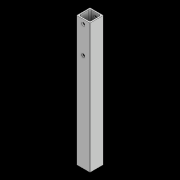
# Autodesk Inventor part: am-3594 5-8x5-8 0.063 wall tubing
Saved by Autodesk Inventor 2022 (Build 260153000, 153)
## iProperties
Created: 2021-10-09
Part Number: am-3594 5-8x5-8 0.063 wall tubing
Material: Generic
Document SubType Name: Modeling
Designer: timmy
Density: 1 g/cm^3
Appearance: Default
Author: timmy
Autodesk Inventor part; units mm, degrees
ref_plane "YZ Plane" through (0, 0, 0) normal (1, 0, 0) x (0, 1, 0)
ref_plane "XZ Plane" through (0, 0, 0) normal (0, 1, 0) x (-1, 0, 0)
ref_plane "XY Plane" through (0, 0, 0) normal (0, 0, 1) x (1, 0, 0)
sketch "Sketch1" plane through (0, 0, 0) normal (0, 1, 0) x (-1, 0, 0)
  line L0 (0, 0) -> (-15.875, 0)
  line L1 (-15.875, 0) -> (-15.875, -15.875)
  line L2 (-15.875, -15.875) -> (0, -15.875)
  line L3 (0, -15.875) -> (0, 0)
  dimension "d0" = 15.875
  dimension "d1" = 15.875
  constraints: 8 end point, 2 parallel, 1 horizontal, 1 perpendicular
  measures "d0" distance of L2.end L1.end
  measures "d1" distance of L1.end L0.end
extrude "Extrusion1" add sketch "Sketch1" along normal blind 152.4
sketch "Sketch2" plane through (0, 0, 0) normal (0, -1, 0) x (1, 0, 0)
  line L0 (15.875, 0) -> (15.875, -15.875) projected
  line L1 (0, 0) -> (15.875, 0) projected
  line L2 (0, -15.875) -> (0, 0) projected
  line L3 (15.875, -15.875) -> (0, -15.875) projected
  line L4 (14.2748, -14.2748) -> (14.2748, -1.6002)
  line L5 (14.2748, -1.6002) -> (1.6002, -1.6002)
  line L6 (1.6002, -1.6002) -> (1.6002, -14.2748)
  line L7 (1.6002, -14.2748) -> (14.2748, -14.2748)
  dimension "d4" = 1.6002
  constraints: 8 end point, 3 other
  measures "d4" distance between parallel lines of L0 L4
extrude "Extrusion2" cut sketch "Sketch2" against normal blind 152.4 contours L7 L6 L5 L4
fillet "Fillet1" radius 1.524 4 edges at (14.2748, 76.2, -14.2748) (1.6002, 76.2, -1.6002) (14.2748, 76.2, -1.6002) (1.6002, 76.2, -14.2748)
fillet "Fillet2" radius 0.254 4 edges at (15.875, 76.2, 0) (15.875, 76.2, -15.875) (0, 76.2, -15.875) (0, 76.2, 0)
sketch "Sketch3" plane through (0.254, 0, 0) normal (0, 0, 1) x (1, 0, 0)
  line L0 (15.367, 152.4) -> (0, 152.4) projected
  line L1 (7.6835, 152.4) -> (7.6835, 147.32)
  circle A0 centre (7.6835, 147.32) radius 1.905
  point P0 (-0.254, 0)
  dimension "d9" = 5.08
  dimension "d10" = 3.81
  constraints: 2 end point, 1 centre point, 1 coincident, 1 midpoint, 1 vertical
  measures "d9" distance of L1.start L1.end
  measures "d10" diameter of A0
extrude "Extrusion3" cut sketch "Sketch3" against normal blind 15.875
sketch "Sketch4" plane through (0.254, 0, 0) normal (0, 0, 1) x (1, 0, 0)
  circle A0 centre (7.6835, 147.32) radius 1.905 projected
  line L0 (7.6835, 147.32) -> (7.6835, 117.221)
  circle A1 centre (7.6835, 115.316) radius 1.905
  point P0 (-0.254, 0)
  dimension "d13" = 30.099
  constraints: 2 end point, 1 vertical, 1 vertical alignment, 2 other
  measures "d13" distance of L0.start L0.end
extrude "Extrusion4" cut sketch "Sketch4" against normal blind 15.875 contours A1
body "Solid1"
